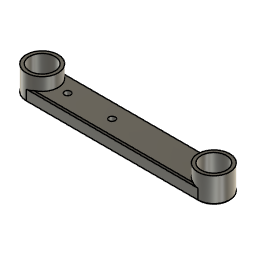
Motor Plate v6 (Autodesk Fusion 360 design; units mm, degrees)
Autodesk Fusion 360 part; units mm, degrees
sketch "Sketch1" plane through (0, 0, 0) normal (0, 0, 1) x (1, 0, 0)
  circle A0 centre (0, 0) radius 10
  circle A1 centre (0, 0) radius 12.5
  line L0 (0, 0) -> (135, 0) construction
  circle A2 centre (135, 0) radius 10
  circle A3 centre (135, 0) radius 12.5
  line L1 (0, 12.5) -> (135, 12.5)
  line L2 (0, -12.5) -> (135, -12.5)
  circle A4 centre (20, 0) radius 2.5
  circle A5 centre (55, 0) radius 2.5
  circle A6 centre (0, 0) radius 1.5
  circle A7 centre (135, 0) radius 1.5
  dimension "d1" = 20
  dimension "d2" = 25
  dimension "d3" = 20
  dimension "d5" = 135
  dimension "d6" = 5
  dimension "d7" = 5
  dimension "d8" = 35
  dimension "d9" = 20
  dimension "d16" = 3
  dimension "d17" = 3
  constraint coincident A0.centre A1.centre
  constraint concentric A0 A1
  constraint horizontal L0
  constraint coincident L0.end A2.centre
  constraint concentric A2 A3
  constraint coincident A1 L1.start
  constraint coincident A3 L1.end
  constraint tangent A3 L1
  constraint horizontal L1
  constraint coincident A1 L2.start
  constraint coincident A3 L2.end
  constraint tangent A3 L2
  constraint parallel L1 L2
  constraint coincident L0 A4.centre
  constraint coincident L0 A5.centre
  constraint concentric A2 A7
  constraint equal A1 A3
  measures "d1" diameter of A0
  measures "d2" diameter of A1
  measures "d3" diameter of A2
  measures "d5" distance of A0.centre L0.end
  measures "d6" diameter of A4
  measures "d7" diameter of A5
  measures "d8" distance of A4.centre A5.centre
  measures "d9" distance of A0.centre A4.centre
  measures "d16" diameter of A6
  measures "d17" diameter of A7
extrude "Extrude1" add sketch "Sketch1" along normal blind 10 contours A1 A3 L1 L2 makes body 1
extrude "Extrude2" add sketch "Sketch1" along normal blind 5 separate body contours A0 | A2 | A6 | A7 makes body 2 at (9.9876, -0.4985, 3.3333) makes body 3 at (131.9968, 2.3092, 0)
extrude "Extrude3" add sketch "Sketch1" along normal blind 20 contours A1 | A3 bodies 1 2 3
extrude "Extrude4" cut sketch "Sketch1" along normal through all contours A6 | A7 bodies 1
chamfer "Chamfer1" distance 1 angle 45 1 faces at (108.6406, -4.5163, 0) on bodies 1
chamfer "Chamfer2" distance 1 angle 45 2 edges at (67.5, 12.5, 10) (67.5, -12.5, 10) on bodies 1
